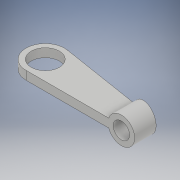
# Autodesk Inventor part: motor test flapper nema23
Saved by Autodesk Inventor 2018.2 (Build 222227000, 227)
## iProperties
Created: 2018-03-04
Part Number: motor test flapper nema23
Material: Generic
Document SubType Name: Modeling
Designer: torba
Density: 1 g/cm^3
Appearance: Default
Author: torba
Autodesk Inventor part; units mm, degrees
ref_plane "YZ Plane" through (0, 0, 0) normal (1, 0, 0) x (0, 1, 0)
ref_plane "XZ Plane" through (0, 0, 0) normal (0, 1, 0) x (-1, 0, 0)
sketch "Sketch11" plane through (0, 0, 0) normal (0, 1, 0) x (-1, 0, 0)
  circle A0 centre (-0.0131, -0.1514) radius 8.2
  line L0 (-60.521, -4.7173) -> (-51.406, -3.2969)
  circle A1 centre (-0.0131, -0.1514) radius 11.2
  line L1 (-51.406, -3.2969) -> (-48.4439, -3.7726)
  line L2 (-60.521, -4.7173) -> (-63.5128, -4.9389)
  line L3 (-48.4439, -3.7726) -> (-1.7762, -11.2118)
  line L4 (-48.4439, -3.7726) -> (-50.7535, 11.0486)
  line L5 (-50.7535, 11.0486) -> (-0.0131, 11.0486)
  line L6 (-78.4528, 0) -> (26.1269, 0) projected
  point P0 (0, 0)
  point P1 (-59.9072, 24.0613)
  point P2 (-55.9635, -4.0071)
  dimension "d63" = 16.4
  dimension "d64" = 22.4
  dimension "d65" = 9.225
  dimension "d66" = 3
  dimension "d67" = 3
  dimension "d68" = 15
  dimension "d77" = 48.4109
  dimension "d78" = 9.057
  dimension "d79" = 8.857
  dimension "d80" = 11.0486
  dimension "d81" = 11.3516
  dimension "d82" = 13.0128
  dimension "d83" = 25.6823
  constraints: 12 end point, 2 centre point, 2 point on circle, 2 tangent, 1 coincident, 1 midpoint, 1 parallel
  measures "d63" diameter of A0
  measures "d64" diameter of A1
  measures "d65" distance of L0.start L0.end
  measures "d66" distance of L0.end L1.end
  measures "d67" distance of L0.start L2.end
  measures "d68" distance of L1.end L4.end
  measures "d77" distance from line of A0.centre L4
  measures "d78" angle of L5 L3
  measures "d79" angle of L0 L5
  measures "d80" distance from line of point (0, 0) L5
  measures "d81" distance from line of point (0, 0) L3
  measures "d82" distance from line of point (-59.907, 24.061) L5
  measures "d83" distance from line of point (-59.907, 24.061) L3
extrude "Extrusion9" add sketch "Sketch11" along normal blind 5 contours A0 L6 A1 | A0 L6 A1 | L6 L4 L5 A1 | A1 L3 L4 L6
ref_plane "Work Plane2" through (0, 0, 0) normal (0, 0, 1) x (1, 0, 0)
sketch "Sketch12" plane through (0, 0, 0) normal (0, 0, 1) x (1, 0, 0)
  line L0 (48.4439, 0) -> (48.4439, 5) projected
  line L1 (48.4439, 0) -> (1.7762, 0) projected
  line L2 (48.4439, 0) -> (1.7762, 0) projected
  line L3 (1.7762, 0) -> (1.7762, 5) projected
  line L4 (48.4439, 5) -> (1.7762, 5) projected
  line L5 (48.4439, 0) -> (48.4439, 5) projected
  line L6 (50.7535, 0) -> (50.7535, 5) projected
  line L7 (50.7535, 2.5) -> (55.5165, 2.5)
  circle A0 centre (55.5165, 2.5) radius 4.763
  circle A1 centre (55.5165, 2.5) radius 7.763
  point P0 (0, 0)
  dimension "d72" = 4.763
  dimension "d73" = 15.526
  constraints: 2 coincident, 2 end point, 1 centre point, 1 horizontal, 1 horizontal alignment, 4 other
  measures "d72" distance of L7.start L7.end
  measures "d73" diameter of A1
extrude "Extrusion10" add sketch "Sketch12" along normal up to surface contours L1 A1 L4 L0 | L0 L4 A1 L1 starts on plane at (48.4439, 0, -3.7726) facing (0.1574204, 0, -0.9875317) surface through (0.0131, 0, 11.0486) normal (0, 0, 1)
body "Solid3"
